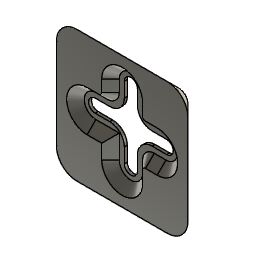
Model_Bracket (Autodesk Fusion 360 design; units mm, degrees)
Autodesk Fusion 360 part; units mm, degrees
note: some values were not read from the file. Set by a fixed rule: which sketch regions a step uses.
sketch "Sketch2" plane through (0, 0, 0) normal (0, 1, 0) x (1, 0, 0)
  line L0 (22.5, -22.5) -> (-22.5, -22.5)
  line L1 (-22.5, -22.5) -> (-22.5, 22.5)
  line L2 (-22.5, 22.5) -> (22.5, 22.5)
  line L3 (22.5, 22.5) -> (22.5, -22.5)
  dimension "d7" = 45
  dimension "d8" = 45
  dimension "d23" = 22.5
  dimension "d24" = 22.5
  constraint horizontal L0
  constraint vertical L1
  constraint horizontal L2
  constraint vertical L3
  measures "d7" distance of L0.start L0.end
  measures "d8" distance of L0.end L1.end
  measures "d23" distance of origin L1
  measures "d24" distance of origin L0
extrude "Extrude4" add sketch "Sketch2" along normal blind 4
sketch "Sketch5" plane through (0, 0, 0) normal (0, 1, 0) x (1, 0, 0)
  line L0 (-2.25, -7.25) -> (-2.25, -12.25)
  line L1 (2.25, -12.25) -> (2.25, -7.25)
  line L2 (7.25, -2.25) -> (12.25, -2.25)
  line L3 (7.25, 2.25) -> (12.25, 2.25)
  line L4 (2.25, 7.25) -> (2.25, 12.25)
  line L5 (-2.25, 7.25) -> (-2.25, 12.25)
  line L6 (-7.25, 2.25) -> (-12.25, 2.25)
  line L7 (-7.25, -2.25) -> (-12.25, -2.25)
  arc A0 (-2.25, -12.25) -> (2.25, -12.25) centre (0, -12.25) ccw
  arc A1 (12.25, -2.25) -> (12.25, 2.25) centre (12.25, 0) ccw
  arc A2 (2.25, 12.25) -> (-2.25, 12.25) centre (0, 12.25) ccw
  arc A3 (-12.25, 2.25) -> (-12.25, -2.25) centre (-12.25, 0) ccw
  arc A4 (-2.25, -7.25) -> (-7.25, -2.25) centre (-7.25, -7.25) ccw
  arc A5 (-7.25, 2.25) -> (-2.25, 7.25) centre (-7.25, 7.25) ccw
  arc A6 (7.25, -2.25) -> (2.25, -7.25) centre (7.25, -7.25) ccw
  arc A7 (2.25, 7.25) -> (7.25, 2.25) centre (7.25, 7.25) ccw
  point P0 (-2.25, -2.25)
  point P1 (2.25, -2.25)
  point P2 (2.25, 2.25)
  point P3 (-2.25, 2.25)
  dimension "d29" = 10
  dimension "d30" = 2.25
  dimension "d32" = 4.5
  dimension "d33" = 10
  dimension "d35" = 2.25
  dimension "d36" = 2.25
  dimension "d37" = 10
  dimension "d38" = 4.5
  dimension "d39" = 2.25
  dimension "d40" = 10
  dimension "d41" = 4.5
  dimension "d54" = 4.5
  dimension "d56" = 10
  dimension "d57" = 10
  dimension "d58" = 10
  dimension "d59" = 10
  dimension "d61" = 5
  constraint vertical L0
  constraint vertical L1
  constraint perpendicular L1 L2
  constraint horizontal L3
  constraint perpendicular L3 L4
  constraint vertical L5
  constraint perpendicular L5 L6
  constraint perpendicular L0 L7
  constraint tangent L1 A0
  constraint tangent L3 A1
  constraint tangent L5 A2
  constraint tangent L6 A3
  constraint coincident P0 L0
  constraint coincident P0 L7
  constraint tangent L0 A4
  constraint tangent L7 A4
  constraint coincident P3 L5
  constraint coincident P3 L6
  constraint tangent L5 A5
  constraint tangent L6 A5
  constraint equal A4 A5
  constraint coincident P1 L1
  constraint coincident P1 L2
  constraint tangent L1 A6
  constraint tangent L2 A6
  constraint equal A4 A6
  constraint coincident P2 L3
  constraint coincident P2 L4
  constraint tangent L3 A7
  constraint tangent L4 A7
  constraint equal A4 A7
  measures "d29" distance of P0 L0.end
  measures "d30" distance of L0 origin
  measures "d32" distance of L0 L1
  measures "d33" distance of L1.start P1
  measures "d35" vertical distance of P0 origin
  measures "d36" vertical distance of origin P1
  measures "d37" distance of P1 L2.end
  measures "d38" distance of L2 L3
  measures "d39" horizontal distance of origin P2
  measures "d40" distance of P2 L4.end
  measures "d41" distance of L4 L5
  measures "d54" distance of L6 L7
  measures "d56" distance of P2 L3.end
  measures "d57" distance of P0 L7.end
  measures "d58" distance of P3 L6.end
  measures "d59" distance of P3 L5.end
  measures "d61" radius of A4
extrude "Extrude5" cut sketch "Sketch5" along normal blind 5
sketch "Sketch7" plane through (0, 0, 0) normal (0, 1, 0) x (1, 0, 0)
  line L0 (-7, -8) -> (-7, -12)
  line L1 (-8, -7) -> (-12, -7)
  line L2 (8, -7) -> (12, -7)
  line L3 (7, -8) -> (7, -12)
  line L4 (7, 8) -> (7, 12)
  line L5 (8, 7) -> (12, 7)
  line L6 (-7, 7) -> (-12, 7)
  line L7 (-7, 7) -> (-7, 12)
  arc A0 (-7, -12) -> (7, -12) centre (0, -12) ccw
  arc A1 (12, -7) -> (12, 7) centre (12, 0) ccw
  arc A2 (7, 12) -> (-7, 12) centre (0, 12) ccw
  arc A3 (-12, 7) -> (-12, -7) centre (-12, 0) ccw
  arc A4 (8, -7) -> (7, -8) centre (8, -8) ccw
  arc A5 (7, 8) -> (8, 7) centre (8, 8) ccw
  arc A6 (-7, -8) -> (-8, -7) centre (-8, -8) ccw
  point P0 (-7, -7)
  dimension "d63" = 5
  dimension "d64" = 5
  dimension "d65" = 7
  dimension "d66" = 7
  dimension "d69" = 1
  constraint vertical L0
  constraint perpendicular L0 L1
  constraint tangent L3 A0
  constraint tangent L5 A1
  constraint tangent L4 A2
  constraint tangent L6 A3
  constraint tangent L2 A4
  constraint tangent L3 A4
  constraint tangent L4 A5
  constraint tangent L5 A5
  constraint equal A4 A5
  constraint coincident P0 L0
  constraint coincident P0 L1
  constraint tangent L0 A6
  constraint tangent L1 A6
  constraint equal A4 A6
  measures "d63" distance of P0 L0.end
  measures "d64" distance of P0 L1.end
  measures "d65" distance of origin L0
  measures "d66" distance of origin L1
  measures "d69" radius of A4
extrude "Extrude7" cut sketch "Sketch7" along normal blind 3
chamfer "Chamfer2" distance 3 angle 45 15 edges at (-9.5, 3, -7) (-19, 3, 0) (-10, 3, 7) (-7.2929, 3, 7.2929) (-7, 3, 10) (0, 3, 19) (7, 3, 10) (7.2929, 3, 7.2929) (10, 3, 7) (19, 3, 0) (10, 3, -7) (7.2929, 3, -7.2929) (7, 3, -10) (0, 3, -19) (-7, 3, -9.5)
fillet "Fillet1" radius 7 4 edges at (-22.5, 2, 22.5) (-22.5, 2, -22.5) (22.5, 2, -22.5) (22.5, 2, 22.5)
chamfer "Chamfer3" distance 4 angle 45 8 edges at (0, 4, -22.5) (20.4497, 4, -20.4497) (22.5, 4, 0) (20.4497, 4, 20.4497) (0, 4, 22.5) (-20.4497, 4, 20.4497) (-22.5, 4, 0) (-20.4497, 4, -20.4497)
